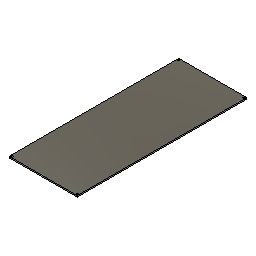
liteboard-backplane (Autodesk Fusion 360 design; units mm, degrees)
part number: 2026-04-13-21-45-43-966
Autodesk Fusion 360 part; units mm, degrees
sketch "草图1" plane through (0, 0, 0) normal (0, 0, 1) x (1, 0, 0)
  line L0 (48.1, -119.85) -> (-48.1, -119.85)
  line L1 (-48.1, -119.85) -> (-48.1, 119.85)
  line L2 (-48.1, 119.85) -> (48.1, 119.85)
  line L3 (48.1, 119.85) -> (48.1, -119.85)
  line L4 (48.1, -119.85) -> (-48.1, 119.85) construction
  line L5 (-48.1, -119.85) -> (48.1, 119.85) construction
  dimension "d1" = 96.2
  dimension "d2" = 239.7
  constraint horizontal L0
  constraint perpendicular L0 L1
  constraint parallel L0 L2
  constraint parallel L1 L3
  constraint coincident L4 origin
  constraint coincident L5 origin
  measures "d1" distance of L1.end L2.end
  measures "d2" distance of L0.end L1.end
extrude "拉伸1" add sketch "草图1" along normal blind 2.5 makes body 1
sketch "草图2" plane through (0, 0, 0) normal (0, 0, -1) x (1, 0, 0)
  line L0 (-48.1, -119.85) -> (48.1, -119.85)
  line L1 (48.1, -119.85) -> (48.1, 119.85)
  line L2 (48.1, 119.85) -> (-48.1, 119.85)
  line L3 (-48.1, 119.85) -> (-48.1, -119.85)
  circle A0 centre (-46.5, -118) radius 1.25
  circle A1 centre (-46.5, 118) radius 1.25
  circle A2 centre (46.5, 118) radius 1.25
  circle A3 centre (46.5, -118) radius 1.25
  dimension "d5" = 2.5
  dimension "d6" = 2.5
  dimension "d7" = 2.5
  dimension "d8" = 2.5
  measures "d5" diameter of A0
  measures "d6" diameter of A1
  measures "d7" diameter of A2
  measures "d8" diameter of A3
extrude "拉伸2" cut sketch "草图2" against normal blind 0.9 contours A0 | A1 | A2 | A3 bodies 1
imported_body "衍生的基础特征1" makes body 2
move_body "移动1" bodies 2 to x (0, -1, 0) y (1, 0, 0) z (0, 0, 1) at (43.6318, 106.1995, 0)
extrude "拉伸3" add sketch "草图2" against normal blind 0.5 contours A0 | A1 | A2 | A3 bodies 1
sketch "草图3" plane through (0, 0, 0) normal (0, 0, -1) x (1, 0, 0)
  line L0 (-48.1, -119.85) -> (48.1, -119.85)
  line L1 (48.1, -119.85) -> (48.1, 119.85)
  line L2 (48.1, 119.85) -> (-48.1, 119.85)
  line L3 (-48.1, 119.85) -> (-48.1, -119.85)
  circle A0 centre (46.1352, -117.7022) radius 1.2483
  circle A1 centre (-45.869, -117.6978) radius 1.25
  circle A2 centre (-45.8604, 117.8069) radius 1.25
  circle A3 centre (46.1314, 117.807) radius 1.25
  dimension "d21" = 2.5
  dimension "d22" = 2.5
  dimension "d23" = 2.5
  measures "d21" diameter of A1
  measures "d22" diameter of A2
  measures "d23" diameter of A3
extrude "拉伸4" cut sketch "草图3" against normal blind 5 contours A0 | A1 | A2 | A3 bodies 1
fillet "圆角5" radius 0.7 2 edges at (0, 119.85, 0) (48.1, 0, 0) on bodies 1
fillet "圆角6" radius 0.7 6 edges at (48.1, -119.85, 1.6) (47.895, -119.85, 0.205) (-0.35, -119.85, 0) (-48.1, -0.35, 0) (-48.1, 119.645, 0.205) (-48.1, 119.85, 1.6) on bodies 1
delete_body "移除实体1" bodies 2
named bodies: "实体2"
